果盘附件 (Autodesk Fusion 360 design; units mm, degrees)
part number: 2026-02-27-15-44-32-501
Autodesk Fusion 360 part; units mm, degrees
sketch "草图1" plane through (0, 0, 0) normal (0, 0, 1) x (1, 0, 0)
  circle A0 centre (0, 0) radius 34.25
  circle A1 centre (0, 0) radius 32.75
  dimension "d1" = 68.5
  dimension "d2" = -1.5
  constraint coincident A0.centre A1.centre
  measures "d1" diameter of A0
extrude "拉伸1" add sketch "草图1" along normal blind 1.5 contours A0 | A1 makes body 1
extrude "拉伸2" cut sketch "草图1" along normal blind 40 bodies 1
extrude "拉伸3" add sketch "草图1" along normal blind 57 bodies 1
ref_plane "工作平面1" through (18, 0, 0) normal (1, 0, 0) x (0, 1, 0)
sketch "草图3" plane through (18, 0, 0) normal (1, 0, 0) x (0, 1, 0)
  arc A0 (6.4, 57.6) -> (-6.4, 57.6) centre (0, 52.8) ccw
  arc A1 (4.8, 56.4) -> (6.4, 57.6) centre (5.6, 57) ccw
  arc A2 (4.8, 56.4) -> (-4.8, 56.4) centre (0, 52.8) ccw
  arc A3 (-6.4, 57.6) -> (-4.8, 56.4) centre (-5.6, 57) ccw
  arc A4 (5.6, 57) -> (-5.6, 57) centre (0, 52.8) ccw construction
  line L0 (34.25, 57) -> (-34.25, 57)
  line L1 (34.25, 0) -> (-34.25, 0)
  line L2 (0, 0) -> (0, 67.7066) construction
  dimension "d22" = 7
  dimension "d23" = 8
  dimension "d24" = 6
  dimension "d25" = 11.2
  constraint tangent A0 A1
  constraint tangent A1 A2
  constraint tangent A2 A3
  constraint tangent A0 A3
  constraint coincident A1.centre L0
  constraint coincident L2.start origin
  constraint vertical L2
  constraint coincident A0.centre L2
  constraint coincident A3.centre L0
  measures "d22" distance of A1.centre A0.centre
  measures "d23" radius of A0
  measures "d24" radius of A2
  measures "d25" distance of A3.centre A1.centre
extrude "拉伸5" add sketch "草图3" along normal blind 18 separate body contours A0 A1 A2 A3 L0 makes body 2
extrude "拉伸7" cut 1 faces at (33.6225, -1.7016, 57) along direction (0, 0, 1) blind 10 keep common part on bodies 1 bodies 2
pattern_circular "C-阵列2" count 2 over 360 about axis through (0, 0, 1.75) along (0, 0, 1) of bodies 2 makes body 3
